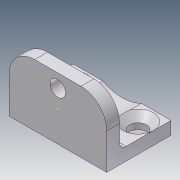
# Autodesk Inventor part: J005359
Saved by Autodesk Inventor 2015 SP1 (Build 190203100, 203)
## iProperties
Created: 2015-08-10
Material: ALUMINUM, 6061-T651
Vendor: HHMI: JRC - ID&F
Document SubType Name: Modeling
Designer: ARNOLDJ
Density: 2.7 g/cm^3
Appearance: Metal-AL-6061 (Machined)
Part Number: J005359
Description: EM MOUNT FOR ROTARY LOCK
Project: P-201804
RuleStatus: InUse
AfterDocSave0: file://Part Number Cleaner
LAB/DEPT: SVOBODA (LAB)
REQUESTING SCIENTIST: SOFRONIEW, NICK
SURFACE ROUGHNESS: 63 Ra
DESIGN DEPARTMENT: HHMI: JRC - ID&F
SPECIAL FINISH: NONE
ALTERED ITEM PART NUMBER: N/A
ALTERED ITEM VENDOR: N/A
ALTERED ITEM DESCRIPTION: N/A
Author: ARNOLDJ
Revision Number: -
Autodesk Inventor part; units mm, degrees
ref_plane "YZ Plane" through (0, 0, 0) normal (1, 0, 0) x (0, 1, 0)
ref_plane "XZ Plane" through (0, 0, 0) normal (0, 1, 0) x (-1, 0, 0)
ref_plane "XY Plane" through (0, 0, 0) normal (0, 0, 1) x (1, 0, 0)
sketch "Sketch1" plane through (0, 0, 0) normal (0, 0, 1) x (1, 0, 0)
  line L0 (12.065, -7.62) -> (-12.065, -7.62)
  line L1 (-12.065, -7.62) -> (-12.065, 7.62)
  line L2 (-12.065, 7.62) -> (12.065, 7.62)
  line L3 (12.065, 7.62) -> (12.065, -7.62)
  line L4 (12.065, -7.62) -> (-12.065, 7.62) construction
  line L5 (-12.065, -7.62) -> (12.065, 7.62) construction
  point P0 (0, 0)
  dimension "d0" = 24.13
  dimension "d1" = 15.24
  constraints: 12 end point, 2 midpoint, 2 parallel, 1 horizontal, 1 perpendicular
  measures "d0" distance of L1.end L2.end
  measures "d1" distance of L0.end L1.end
extrude "Extrusion1" add sketch "Sketch1" along normal blind 3.175
sketch "Sketch2" plane through (0, 0, 0) normal (0, 0, 1) x (1, 0, 0)
  line L0 (12.065, 7.62) -> (12.065, -7.62) projected
  line L1 (-12.065, -7.62) -> (-12.065, 7.62) projected
  line L2 (12.065, -7.62) -> (-12.065, -7.62) projected
  line L3 (12.065, -7.62) -> (-12.065, -7.62)
  line L4 (-12.065, -7.62) -> (-12.065, -4.445)
  line L5 (-12.065, -4.445) -> (12.065, -4.445)
  line L6 (12.065, -4.445) -> (12.065, -7.62)
  point P0 (0, 0)
  dimension "d4" = 3.175
  constraints: 8 end point, 2 parallel, 1 horizontal, 1 perpendicular, 1 point on line
  measures "d4" distance between parallel lines of L2 L5
extrude "Extrusion2" add sketch "Sketch2" against normal blind 12.7
sketch "Sketch3" plane through (-12.065, -4.445, 0) normal (0, 1, 0) x (1, 0, 0)
  line L0 (0, 0) -> (24.13, 0) projected
  line L1 (12.065, 0) -> (12.065, 12.7) construction
  line L2 (24.13, 12.7) -> (0, 12.7) projected
  line L3 (24.13, -3.175) -> (0, -3.175) projected
  point P0 (3.81, 8.382)
  point P1 (20.32, 8.382)
  point P2 (3.81, -6.5118)
  point P3 (20.32, -6.5118)
  dimension "d34" = 16.51
  dimension "d35" = 8.255
  dimension "d37" = 11.557
  constraints: 2 end point, 2 horizontal alignment, 2 midpoint, 2 vertical alignment
  measures "d34" distance of point (20.32, 8.382) point (3.81, 8.382)
  measures "d35" distance from line of L1 point (3.81, 8.382)
  measures "d37" distance from line of L3 point (3.81, 8.382)
hole "Hole1" at (-8.255, -4.445, -8.382) at (8.255, -4.445, -8.382) direction (0, -1, 0) diameter 4.191 end through all countersink diameter 7.62 countersink angle 90
sketch "Sketch4" plane through (0, 0, 3.175) normal (0, 0, 1) x (1, 0, 0)
  point P0 (0, 0)
sketch "Sketch5" plane through (0, 0, 3.175) normal (0, 0, 1) x (1, 0, 0)
  line L0 (-12.065, -7.62) -> (12.065, -7.62) projected
  line L1 (12.065, 7.62) -> (-12.065, 7.62) projected
  point P0 (0, 0)
  point P1 (0, 4.318)
  dimension "d18" = 11.938
  dimension "d27" = 3.302
  measures "d18" distance from line of L0 point (0, 4.318)
  measures "d27" distance from line of point (0, 4.318) L1
hole "Hole2" at (0, 4.318, 3.175) direction (0, 0, -1) diameter 3.7973 end through all
fillet "Fillet2" radius 1.5875 1 edges at (0, -4.445, 0)
fillet "Fillet1" radius 6.35 2 edges at (12.065, 7.62, 1.5875) (-12.065, 7.62, 1.5875)
sketch "Sketch6" plane through (0, 0, 0) normal (0, 0, -1) x (-1, 0, 0)
  circle A0 centre (0, 4.318) radius 1.8986 projected
  line L0 (12.065, -4.445) -> (-12.065, -4.445) projected
  circle A1 centre (0, 4.699) radius 10.3124
  circle A2 centre (0, 4.318) radius 9.9187 construction
  circle A3 centre (0, 4.318) radius 9.525 construction
  point P0 (0, 0)
  dimension "d38" = 20.6248
  dimension "d39" = 0.381
  dimension "d40" = 19.8374
  dimension "d41" = 19.05
  constraints: 3 centre point, 2 coincident
  measures "d38" diameter of A1
  measures "d39" distance of A0.centre A1.centre
  measures "d40" diameter of A2
  measures "d41" diameter of A3
extrude "Extrusion3" cut sketch "Sketch6" along normal up to surface (12.7 mm away)
sketch "Sketch7" plane through (12.065, -4.445, -1.5875) normal (0, 1, 0) x (1, 0, 0)
  circle A0 centre (-20.32, 6.6675) radius 1.2319 projected
  point P0 (-12.065, -1.5875)
equation "\"d35\" = 0.5 * d34"
body "Solid1"
